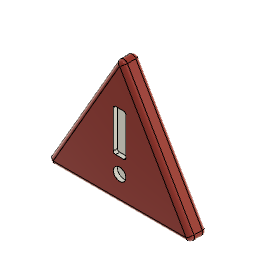
ErrorSign (Autodesk Fusion 360 design; units mm, degrees)
Autodesk Fusion 360 part; units mm, degrees
sketch "Sketch1" plane through (0, 0, 0) normal (0, 1, 0) x (1, 0, 0)
  line L0 (2.1979, -3.8094) -> (42.6124, -73.8552)
  line L1 (47.0126, -73.8552) -> (87.4271, -3.8094)
  line L2 (85.227, 0) -> (4.398, 0)
  arc A0 (42.6124, -73.8552) -> (47.0126, -73.8552) centre (44.8125, -72.5858) ccw
  arc A1 (87.4271, -3.8094) -> (85.227, 0) centre (85.227, -2.54) ccw
  arc A2 (4.398, 0) -> (2.1979, -3.8094) centre (4.398, -2.54) ccw
  dimension "d1" = 2.54
  dimension "d2" = 2.54
  constraint horizontal L2
  constraint tangent L0 A0
  constraint tangent L1 A0
  constraint tangent L1 A1
  constraint tangent L2 A1
  constraint equal A0 A1
  constraint tangent L0 A2
  constraint tangent L2 A2
  measures "d1" radius of A0
  measures "d2" radius of A2
extrude "Extrude1" add sketch "Sketch1" along normal blind 10.16
sketch "Sketch2" plane through (0, 0, 0) normal (0, -1, 0) x (1, 0, 0)
  arc A0 (2.1979, 3.8094) -> (4.398, 0) centre (4.398, 2.54) ccw
  line L0 (4.398, 0) -> (85.227, 0)
  arc A1 (85.227, 0) -> (87.4271, 3.8094) centre (85.227, 2.54) ccw
  line L1 (87.4271, 3.8094) -> (47.0126, 73.8552)
  arc A2 (47.0126, 73.8552) -> (42.6124, 73.8552) centre (44.8125, 72.5858) ccw
  line L2 (42.6124, 73.8552) -> (2.1979, 3.8094)
  circle A3 centre (44.8125, 15.8064) radius 3.81
  line L3 (47.3525, 24.8629) -> (42.2725, 24.8629)
  line L4 (41.0025, 26.1329) -> (41.0025, 48.9929)
  line L5 (42.2725, 50.2629) -> (47.3525, 50.2629)
  line L6 (48.6225, 48.9929) -> (48.6225, 26.1329)
  line L7 (48.6225, 24.8629) -> (41.0025, 50.2629) construction
  line L8 (41.0025, 24.8629) -> (48.6225, 50.2629) construction
  arc A4 (48.6225, 48.9929) -> (47.3525, 50.2629) centre (47.3525, 48.9929) ccw
  arc A5 (42.2725, 50.2629) -> (41.0025, 48.9929) centre (42.2725, 48.9929) ccw
  arc A6 (47.3525, 24.8629) -> (48.6225, 26.1329) centre (47.3525, 26.1329) ccw
  arc A7 (41.0025, 26.1329) -> (42.2725, 24.8629) centre (42.2725, 26.1329) ccw
  point P0 (44.8125, 37.5629)
  dimension "d8" = 7.62
  dimension "d9" = 7.62
  dimension "d10" = 25.4
  dimension "d11" = 1.27
  dimension "d12" = 1.27
  constraint horizontal L3
  constraint perpendicular L3 L4
  constraint parallel L3 L5
  constraint parallel L4 L6
  constraint coincident L7 P0
  constraint coincident L8 P0
  constraint coincident L8.end L5
  constraint coincident L8.end L6
  constraint tangent L5 A4
  constraint tangent L6 A4
  constraint coincident L7.end L5
  constraint coincident L7.end L4
  constraint tangent L5 A5
  constraint tangent L4 A5
  constraint equal A4 A5
  constraint coincident L7.start L6
  constraint coincident L7.start L3
  constraint tangent L6 A6
  constraint tangent L3 A6
  constraint equal A4 A6
  constraint coincident L8.start L3
  constraint coincident L8.start L4
  constraint tangent L3 A7
  constraint tangent L4 A7
  measures "d8" diameter of A3
  measures "d9" distance of L7.end L8.end
  measures "d10" distance of L8.start L7.end
  measures "d11" radius of A4
  measures "d12" radius of A7
extrude "Extrude2" cut sketch "Sketch2" against normal blind 2.54 contours A3 | L3 L4 L5 L6 A4 A5 A6 A7
fillet "Fillet1" radius 2.54 6 edges at (44.8125, 0, 0) (2.1984, 0, 1.2697) (22.4052, 0, 38.8323) (44.8125, 0, 75.1258) (67.2198, 0, 38.8323) (87.4266, 0, 1.2697)
fillet "Fillet2" radius 2.54 6 edges at (44.8125, 10.16, 0) (2.1984, 10.16, 1.2697) (22.4052, 10.16, 38.8323) (44.8125, 10.16, 75.1258) (67.2198, 10.16, 38.8323) (87.4266, 10.16, 1.2697)
